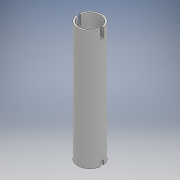
# Autodesk Inventor part: tubo
Saved by Autodesk Inventor 2018 (Build 220112000, 112)
## iProperties
Created: 2020-03-10
Part Number: tubo
Material: Genérico
Document SubType Name: Modeling
Designer: sala.ceri
Density: 1 g/cm^3
Appearance: Valor por defecto
Author: sala.ceri
Autodesk Inventor part; units mm, degrees
ref_plane "YZ Plane" through (0, 0, 0) normal (1, 0, 0) x (0, 1, 0)
ref_plane "XZ Plane" through (0, 0, 0) normal (0, 1, 0) x (-1, 0, 0)
ref_plane "XY Plane" through (0, 0, 0) normal (0, 0, 1) x (1, 0, 0)
sketch "Boceto1" plane through (0, 0, 0) normal (0, 0, 1) x (1, 0, 0)
  circle A0 centre (0, 0) radius 13.175
  circle A1 centre (0, 0) radius 11.5
  dimension "d0" = 26.35
  dimension "d1" = 23
  constraints: 2 centre point, 2 coincident
  measures "d0" diameter of A0
  measures "d1" diameter of A1
extrude "Extrusión1" add sketch "Boceto1" along normal blind 130
sketch "Boceto2" plane through (0, 0, 0) normal (1, 0, 0) x (0, 1, 0)
  line L0 (1.5, 5) -> (1.5, 0)
  line L1 (-13.175, 0) -> (13.175, 0) projected
  line L2 (1.5, 0) -> (-1.5, 0)
  line L3 (-1.5, 0) -> (-1.5, 5)
  line L4 (1.5, 5) -> (-1.5, 5)
  point P0 (0, 0)
  dimension "d6" = 3
  constraints: 8 end point, 2 perpendicular, 1 horizontal, 1 point on line
  measures "d6" distance of L0.end L2.end
extrude "Extrusión2" cut sketch "Boceto2" along normal mid plane 130
sketch "Boceto3" plane through (0, 0, 0) normal (1, 0, 0) x (0, 1, 0)
  line L0 (13.175, 130) -> (-13.175, 130) projected
  line L1 (1.5, 130) -> (-1.5, 130)
  line L2 (1.5, 130) -> (1.5, 120)
  line L3 (1.5, 120) -> (-1.5, 120)
  line L4 (-1.5, 120) -> (-1.5, 130)
  point P0 (0, 0)
  dimension "d10" = 3
  dimension "d11" = 10
  dimension "d12" = 3
  constraints: 8 end point, 2 point on line, 1 perpendicular, 1 vertical
  measures "d10" distance of L1.start L1.end
  measures "d11" distance of L1.start L2.end
  measures "d12" distance of L2.end L3.end
extrude "Extrusión3" cut sketch "Boceto3" along normal mid plane 30
